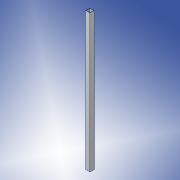
# Autodesk Inventor part: C007
Saved by Autodesk Inventor 2017 (Build 210142000, 142)
## iProperties
Created: 2017-06-14
Part Number: C007
Material: Aluminum 6061
Document SubType Name: Modeling
Designer: zallen
Density: 2.7 g/cm^3
Appearance: Aluminum - Flat
Author: zallen
Autodesk Inventor part; units mm, degrees
ref_plane "YZ Plane" through (0, 0, 0) normal (1, 0, 0) x (0, 1, 0)
ref_plane "XZ Plane" through (0, 0, 0) normal (0, 1, 0) x (-1, 0, 0)
ref_plane "XY Plane" through (0, 0, 0) normal (0, 0, 1) x (1, 0, 0)
sketch "Sketch1" plane through (0, 0, 0) normal (0, 0, 1) x (1, 0, 0)
  line L0 (0, 0) -> (19, 0)
  line L1 (19, 0) -> (19, 600)
  line L2 (19, 600) -> (0, 600)
  line L3 (0, 600) -> (0, 0)
  dimension "d0" = 19
  dimension "d1" = 600
  constraints: 8 end point, 2 parallel, 1 horizontal, 1 perpendicular
  measures "d0" distance of L2.end L1.end
  measures "d1" distance of L1.end L0.end
extrude "Extrusion1" add sketch "Sketch1" along normal blind 19
sketch "Sketch2" plane through (0, 0, 0) normal (0, -1, 0) x (1, 0, 0)
  line L0 (0, 0) -> (0, 19) projected
  line L1 (0, 0) -> (19, 0) projected
  line L2 (19, 0) -> (19, 19) projected
  line L3 (0, 19) -> (19, 19) projected
  line L4 (0, 0) -> (0, 19) projected
  line L5 (17.5, 1.5) -> (1.5, 1.5)
  line L6 (1.5, 1.5) -> (1.5, 17.5)
  line L7 (1.5, 17.5) -> (17.5, 17.5)
  line L8 (17.5, 17.5) -> (17.5, 1.5)
  dimension "d4" = 1.5
  constraints: 8 end point, 3 other
  measures "d4" distance between parallel lines of L1 L5
extrude "Extrusion2" cut sketch "Sketch2" against normal through all contours L5 L6 L7 L8
body "Solid1"
